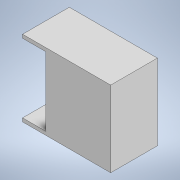
# Autodesk Inventor part: motor_support
Saved by Autodesk Inventor 2022 (Build 260153000, 153)
## iProperties
Created: 2022-01-17
Part Number: motor_support
Material: Generic
Document SubType Name: Modeling
Designer: kylem
Density: 1 g/cm^3
Appearance: Default
Author: kylem
Autodesk Inventor part; units mm, degrees
ref_plane "YZ Plane" through (0, 0, 0) normal (1, 0, 0) x (0, 1, 0)
ref_plane "XZ Plane" through (0, 0, 0) normal (0, 1, 0) x (-1, 0, 0)
ref_plane "XY Plane" through (0, 0, 0) normal (0, 0, 1) x (1, 0, 0)
sketch "Sketch1" plane through (0, 0, 0) normal (0, 1, 0) x (-1, 0, 0)
  line L0 (0, 0) -> (55.38, 0)
  line L1 (55.38, 0) -> (55.38, -40)
  line L2 (55.38, -40) -> (0, -40)
  line L3 (0, -40) -> (0, 0)
  dimension "d0" = 55.38
  dimension "d1" = 40
  constraints: 8 end point, 2 parallel, 1 horizontal, 1 perpendicular
  measures "d0" distance of L1.end L2.end
  measures "d1" distance of L0.end L1.end
extrude "Extrusion1" add sketch "Sketch1" along normal blind 65
sketch "Sketch2" plane through (-55.38, 0, 0) normal (0, 0, 1) x (1, 0, 0)
  line L0 (55.38, 0) -> (0, 0) projected
  line L1 (0, 0) -> (-20, 0)
  line L2 (-20, 0) -> (-20, 3)
  line L3 (-20, 3) -> (0, 3)
  line L4 (0, 3) -> (0, 0)
  line L5 (55.38, 65) -> (0, 65) projected
  line L6 (0, 65) -> (-20, 65)
  line L7 (-20, 65) -> (-20, 62)
  line L8 (-20, 62) -> (0, 62)
  line L9 (0, 62) -> (0, 65)
  dimension "d4" = 20
  dimension "d5" = 3
  dimension "d6" = 20
  dimension "d7" = 3
  constraints: 16 end point, 4 parallel, 2 horizontal, 2 perpendicular
  measures "d4" distance of L2.end L3.end
  measures "d5" distance of L1.end L2.end
  measures "d6" distance of L8.end L7.end
  measures "d7" distance of L7.end L6.end
extrude "Extrusion2" add sketch "Sketch2" against normal blind 40
body "Solid1"
